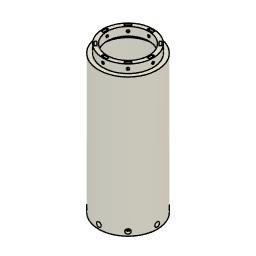
section_fuselage_basique v7 (Autodesk Fusion 360 design; units mm, degrees)
Autodesk Fusion 360 part; units mm, degrees
note: some values were not read from the file. Chosen so that the rebuilt part matches the saved one: which pieces of a blend or face edit are solid.
sketch "Esquisse1" plane through (0, 0, 0) normal (0, 1, 0) x (1, 0, 0)
  circle A0 centre (0, 0) radius 35
  circle A1 centre (0, 0) radius 30
  dimension "d1" = 70
  dimension "d2" = 60
  constraint coincident A0.centre A1.centre
  measures "d1" diameter of A0
  measures "d2" diameter of A1
extrude "Extrusion1" add sketch "Esquisse1" along normal mid plane 150 makes body 1
sketch "Esquisse1 (2)" plane through (0, 0, 0) normal (0, 1, 0) x (1, 0, 0) in component "couplage_standard_femelle v8"
  circle A0 centre (0, 0) radius 35
  circle A1 centre (0, 0) radius 30
  dimension "d1_1" = 70
  dimension "d2_1" = 60
  constraint coincident A0.centre A1.centre
  constraint concentric A0 A1
  measures "d1_1" diameter of A0
  measures "d2_1" diameter of A1
extrude "Extrusion1'" add sketch "Esquisse1 (2)" along normal mid plane 10 separate body makes body 2 in component "couplage_standard_femelle v8"
ref_plane "Plan de construction1" through (35, 0, 0) normal (1, 0, 0) x (0, 1, 0) in component "couplage_standard_femelle v8"
ref_plane "Plan de construction2" through (-35, 0, 0) normal (1, 0, 0) x (0, 1, 0) in component "couplage_standard_femelle v8"
ref_plane "Plan de construction3" through (0, 0, 35) normal (0, 0, 1) x (1, 0, 0) in component "couplage_standard_femelle v8"
ref_plane "Plan de construction4" through (0, 0, -35) normal (0, 0, 1) x (1, 0, 0) in component "couplage_standard_femelle v8"
sketch "Esquisse2" plane through (35, 0, 0) normal (1, 0, 0) x (0, 0, -1) in component "couplage_standard_femelle v8"
  circle A0 centre (0, 0) radius 1.5
  circle A1 centre (0, 0) radius 2.25
  dimension "d9" = 3
  dimension "d10" = 4.5
  constraint coincident A0.centre A1.centre
  constraint concentric A0 A1
  measures "d9" diameter of A0
  measures "d10" diameter of A1
extrude "Extrusion2" cut sketch "Esquisse2" against normal blind 70 contours A0 bodies 2 in component "couplage_standard_femelle v8"
extrude "Extrusion3" cut sketch "Esquisse2" against normal blind 3 bodies 2 in component "couplage_standard_femelle v8"
sketch "Esquisse3" plane through (-35, 0, 0) normal (1, 0, 0) x (0, 0, -1) in component "couplage_standard_femelle v8"
  circle A0 centre (0, 0) radius 2.25
  circle A1 centre (0, 0) radius 1.5
extrude "Extrusion4" cut sketch "Esquisse3" along normal blind 3 bodies 2 in component "couplage_standard_femelle v8"
sketch "Esquisse4" plane through (0, 0, 35) normal (0, 0, 1) x (1, 0, 0) in component "couplage_standard_femelle v8"
  circle A0 centre (0, 0) radius 1.5
  circle A1 centre (0, 0) radius 2.25
  dimension "d17" = 3
  dimension "d18" = 4.5
  constraint coincident A0.centre A1.centre
  measures "d17" diameter of A0
  measures "d18" diameter of A1
extrude "Extrusion5" cut sketch "Esquisse4" against normal blind 70 contours A0 bodies 2 in component "couplage_standard_femelle v8"
extrude "Extrusion6" cut sketch "Esquisse4" against normal blind 3 bodies 2 in component "couplage_standard_femelle v8"
sketch "Esquisse5" plane through (0, 0, -35) normal (0, 0, 1) x (1, 0, 0) in component "couplage_standard_femelle v8"
  circle A0 centre (0, 0) radius 1.5
  circle A1 centre (0, 0) radius 2.25
extrude "Extrusion7" cut sketch "Esquisse5" along normal blind 3 bodies 2 in component "couplage_standard_femelle v8"
move_body "Déplacer1" bodies 2 to x (0.707107, 0, 0.707107) y (0, 1, 0) z (-0.707107, 0, 0.707107) at (0, 0, 0) in component "couplage_standard_femelle v8"
ref_plane "Plan de construction5" through (35, 0, 0) normal (1, 0, 0) x (0, 1, 0) in component "couplage_standard_femelle v8"
ref_plane "Plan de construction6" through (-35, 0, 0) normal (1, 0, 0) x (0, 1, 0) in component "couplage_standard_femelle v8"
ref_plane "Plan de construction7" through (0, 0, 35) normal (0, 0, 1) x (1, 0, 0) in component "couplage_standard_femelle v8"
ref_plane "Plan de construction8" through (0, 0, -35) normal (0, 0, 1) x (1, 0, 0) in component "couplage_standard_femelle v8"
extrude "Extrusion8" cut sketch "Esquisse4" against normal blind 70 contours A0 bodies 2 in component "couplage_standard_femelle v8"
extrude "Extrusion9" cut sketch "Esquisse4" against normal blind 3 bodies 2 in component "couplage_standard_femelle v8"
sketch "Esquisse6" plane through (0, 0, -35) normal (0, 0, 1) x (1, 0, 0) in component "couplage_standard_femelle v8"
  circle A0 centre (0, 0) radius 2.25
  circle A1 centre (0, 0) radius 1.5
extrude "Extrusion10" cut sketch "Esquisse6" along normal blind 3 bodies 2 in component "couplage_standard_femelle v8"
sketch "Esquisse7" plane through (-35, 0, 0) normal (1, 0, 0) x (0, 0, -1) in component "couplage_standard_femelle v8"
  circle A0 centre (0, 0) radius 1.5
  circle A1 centre (0, 0) radius 2.25
  dimension "d35" = 3
  dimension "d36" = 4.5
  constraint coincident A0.centre A1.centre
  measures "d35" diameter of A0
  measures "d36" diameter of A1
extrude "Extrusion11" cut sketch "Esquisse7" along normal blind 70 contours A0 bodies 2 in component "couplage_standard_femelle v8"
extrude "Extrusion12" cut sketch "Esquisse7" along normal blind 3 bodies 2 in component "couplage_standard_femelle v8"
sketch "Esquisse8" plane through (35, 0, 0) normal (1, 0, 0) x (0, 0, -1) in component "couplage_standard_femelle v8"
  circle A0 centre (0, 0) radius 2.25
  circle A1 centre (0, 0) radius 1.5
extrude "Extrusion13" cut sketch "Esquisse8" against normal blind 3 bodies 2 in component "couplage_standard_femelle v8"
move_face "DécalerLesFaces1" offset -0.5 8 faces at (23.3345, 2.25, 23.3345) (33, 2.25, 0) (23.3345, 2.25, -23.3345) (0, 2.25, -33) (-23.3345, 2.25, -23.3345) (-33, 2.25, 0) (-23.3345, 2.25, 23.3345) (0, 2.25, 33) on bodies 2 in component "couplage_standard_femelle v8"
combine "Combiner1" operation add target body 1 tool bodies 2 body 2 seen with x (1, 0, 0) y (0, 1, 0) z (0, 0, 1) at (0, -80, 0)
sketch "Esquisse1 (3)" plane through (0, 0, 0) normal (0, 1, 0) x (1, 0, 0) in component "couplage_standard_male v8"
  circle A0 centre (0, 0) radius 30
  circle A1 centre (0, 0) radius 25
  dimension "d1_2" = 60
  constraint coincident A0.centre A1.centre
  constraint concentric A0 A1
  measures "d1_2" diameter of A0
extrude "Extrusion1''" add sketch "Esquisse1 (3)" along normal mid plane 10 separate body makes body 3 in component "couplage_standard_male v8"
sketch "Esquisse2 (2)" plane through (0, -5, 0) normal (0, -1, 0) x (1, 0, 0) in component "couplage_standard_male v8"
  circle A0 centre (0, 0) radius 25
  circle A1 centre (0, 0) radius 30
  circle A2 centre (0, 0) radius 35
  dimension "d4_2" = 70
  constraint coincident A0.centre A1.centre
  measures "d4_2" diameter of A2
extrude "Extrusion2'" add sketch "Esquisse2 (2)" along normal blind 5 contours A1 | A2 bodies 3 in component "couplage_standard_male v8"
ref_plane "Plan de construction1" through (30, 0, 0) normal (1, 0, 0) x (0, 1, 0) in component "couplage_standard_male v8"
ref_plane "Plan de construction2" through (-30, 0, 0) normal (1, 0, 0) x (0, 1, 0) in component "couplage_standard_male v8"
ref_plane "Plan de construction3" through (0, 0, 30) normal (0, 0, 1) x (1, 0, 0) in component "couplage_standard_male v8"
ref_plane "Plan de construction4" through (0, 0, -30) normal (0, 0, 1) x (1, 0, 0) in component "couplage_standard_male v8"
sketch "Esquisse3 (2)" plane through (30, 0, 0) normal (1, 0, 0) x (0, 0, -1) in component "couplage_standard_male v8"
  circle A0 centre (0, 0) radius 1.5
  dimension "d11_1" = 3
  constraint coincident A0.centre origin
  measures "d11_1" diameter of A0
extrude "Extrusion3'" cut sketch "Esquisse3 (2)" against normal blind 60 bodies 3 in component "couplage_standard_male v8"
sketch "Esquisse4 (2)" plane through (0, 0, -30) normal (0, 0, 1) x (1, 0, 0) in component "couplage_standard_male v8"
  circle A0 centre (0, 0) radius 1.5
  dimension "d14_1" = 3
  constraint coincident A0.centre origin
  measures "d14_1" diameter of A0
extrude "Extrusion4'" cut sketch "Esquisse4 (2)" along normal blind 60 bodies 3 in component "couplage_standard_male v8"
sketch "Esquisse5 (2)" plane through (0, 5, 0) normal (0, 1, 0) x (-1, 0, 0) in component "couplage_standard_male v8"
  circle A0 centre (0, 0) radius 25
  circle A1 centre (0, 0) radius 30
  line L0 (0, 30) -> (0, 25) construction
  line L1 (0, 27.5) -> (-5, 27.5) construction
  line L2 (0, 27.5) -> (5, 27.5) construction
  line L3 (0, 27.5) -> (0, 26.25)
  line L4 (0, 27.5) -> (0, 28.75)
  line L5 (0, 26.25) -> (3.25, 26.25)
  line L6 (0, 28.75) -> (3.25, 28.75)
  line L7 (3.25, 28.75) -> (3.25, 26.25)
  line L8 (0, 26.25) -> (-3.25, 26.25)
  line L9 (0, 28.75) -> (-3.25, 28.75)
  line L10 (-3.25, 28.75) -> (-3.25, 26.25)
  line L11 (-18.5616, 18.5616) -> (-16.2635, 20.8597)
  line L12 (-19.4454, 19.4454) -> (-18.5616, 18.5616)
  line L13 (-19.4454, 19.4454) -> (-20.3293, 20.3293)
  line L14 (-20.3293, 20.3293) -> (-18.0312, 22.6274)
  line L15 (-18.0312, 22.6274) -> (-16.2635, 20.8597)
  line L16 (-18.5616, 18.5616) -> (-20.8597, 16.2635)
  line L17 (-22.6274, 18.0312) -> (-20.8597, 16.2635)
  line L18 (-20.3293, 20.3293) -> (-22.6274, 18.0312)
  line L19 (-19.4454, 19.4454) -> (-22.981, 15.9099) construction
  line L20 (-19.4454, 19.4454) -> (-15.9099, 22.981) construction
  line L21 (-21.2132, 21.2132) -> (-17.6777, 17.6777) construction
  line L22 (-26.25, 0) -> (-26.25, 3.25)
  line L23 (-27.5, 0) -> (-26.25, 0)
  line L24 (-27.5, 0) -> (-28.75, 0)
  line L25 (-28.75, 0) -> (-28.75, 3.25)
  line L26 (-28.75, 3.25) -> (-26.25, 3.25)
  line L27 (-26.25, 0) -> (-26.25, -3.25)
  line L28 (-28.75, -3.25) -> (-26.25, -3.25)
  line L29 (-28.75, 0) -> (-28.75, -3.25)
  line L30 (-27.5, 0) -> (-27.5, -5) construction
  line L31 (-27.5, 0) -> (-27.5, 5) construction
  line L32 (-30, 0) -> (-25, 0) construction
  line L33 (-18.5616, -18.5616) -> (-20.8597, -16.2635)
  line L34 (-19.4454, -19.4454) -> (-18.5616, -18.5616)
  line L35 (-19.4454, -19.4454) -> (-20.3293, -20.3293)
  line L36 (-20.3293, -20.3293) -> (-22.6274, -18.0312)
  line L37 (-22.6274, -18.0312) -> (-20.8597, -16.2635)
  line L38 (-18.5616, -18.5616) -> (-16.2635, -20.8597)
  line L39 (-18.0312, -22.6274) -> (-16.2635, -20.8597)
  line L40 (-20.3293, -20.3293) -> (-18.0312, -22.6274)
  line L41 (-19.4454, -19.4454) -> (-15.9099, -22.981) construction
  line L42 (-19.4454, -19.4454) -> (-22.981, -15.9099) construction
  line L43 (-21.2132, -21.2132) -> (-17.6777, -17.6777) construction
  line L44 (0, -26.25) -> (-3.25, -26.25)
  line L45 (0, -27.5) -> (0, -26.25)
  line L46 (0, -27.5) -> (0, -28.75)
  line L47 (0, -28.75) -> (-3.25, -28.75)
  line L48 (-3.25, -28.75) -> (-3.25, -26.25)
  line L49 (0, -26.25) -> (3.25, -26.25)
  line L50 (3.25, -28.75) -> (3.25, -26.25)
  line L51 (0, -28.75) -> (3.25, -28.75)
  line L52 (0, -27.5) -> (5, -27.5) construction
  line L53 (0, -27.5) -> (-5, -27.5) construction
  line L54 (0, -30) -> (0, -25) construction
  line L55 (18.5616, -18.5616) -> (16.2635, -20.8597)
  line L56 (19.4454, -19.4454) -> (18.5616, -18.5616)
  line L57 (19.4454, -19.4454) -> (20.3293, -20.3293)
  line L58 (20.3293, -20.3293) -> (18.0312, -22.6274)
  line L59 (18.0312, -22.6274) -> (16.2635, -20.8597)
  line L60 (18.5616, -18.5616) -> (20.8597, -16.2635)
  line L61 (22.6274, -18.0312) -> (20.8597, -16.2635)
  line L62 (20.3293, -20.3293) -> (22.6274, -18.0312)
  line L63 (19.4454, -19.4454) -> (22.981, -15.9099) construction
  line L64 (19.4454, -19.4454) -> (15.9099, -22.981) construction
  line L65 (21.2132, -21.2132) -> (17.6777, -17.6777) construction
  line L66 (26.25, 0) -> (26.25, -3.25)
  line L67 (27.5, 0) -> (26.25, 0)
  line L68 (27.5, 0) -> (28.75, 0)
  line L69 (28.75, 0) -> (28.75, -3.25)
  line L70 (28.75, -3.25) -> (26.25, -3.25)
  line L71 (26.25, 0) -> (26.25, 3.25)
  line L72 (28.75, 3.25) -> (26.25, 3.25)
  line L73 (28.75, 0) -> (28.75, 3.25)
  line L74 (27.5, 0) -> (27.5, 5) construction
  line L75 (27.5, 0) -> (27.5, -5) construction
  line L76 (30, 0) -> (25, 0) construction
  line L77 (18.5616, 18.5616) -> (20.8597, 16.2635)
  line L78 (19.4454, 19.4454) -> (18.5616, 18.5616)
  line L79 (19.4454, 19.4454) -> (20.3293, 20.3293)
  line L80 (20.3293, 20.3293) -> (22.6274, 18.0312)
  line L81 (22.6274, 18.0312) -> (20.8597, 16.2635)
  line L82 (18.5616, 18.5616) -> (16.2635, 20.8597)
  line L83 (18.0312, 22.6274) -> (16.2635, 20.8597)
  line L84 (20.3293, 20.3293) -> (18.0312, 22.6274)
  line L85 (19.4454, 19.4454) -> (15.9099, 22.981) construction
  line L86 (19.4454, 19.4454) -> (22.981, 15.9099) construction
  line L87 (21.2132, 21.2132) -> (17.6777, 17.6777) construction
  dimension "d17_1" = 1.25
  dimension "d18_1" = 1.25
  dimension "d19_1" = 3.25
  dimension "d20_1" = 3.25
  dimension "d21_1" = 3.25
  dimension "d25_1" = 360
  constraint coincident A1 L0.start
  constraint coincident A0 L0.end
  constraint vertical L0
  constraint midpoint L0 L1.start
  constraint perpendicular L0 L1
  constraint perpendicular L0 L2
  constraint coincident L0 L3.end
  constraint perpendicular L1 L4
  constraint perpendicular L3 L5
  constraint perpendicular L4 L6
  constraint perpendicular L3 L8
  constraint perpendicular L0 L9
  constraint perpendicular L8 L10
  measures "d17_1" distance of L1.start L3.end
  measures "d18_1" distance of L1.start L4.end
  measures "d19_1" distance of L3.end L5.end
  measures "d20_1" distance of L4.end L6.end
  measures "d21_1" distance of L3.end L8.end
extrude "Extrusion6'" cut sketch "Esquisse5 (2)" against normal blind 8 contours L3 L4 L5 L6 L7 | L3 L4 L8 L9 L10 | L11 L12 L13 L14 L15 | L12 L13 L16 L17 L18 | L22 L23 L24 L25 L26 | L23 L24 L27 L28 L29 | L33 L34 L35 L36 L37 | L34 L35 L38 L39 L40 | L44 L45 L46 L47 L48 | L45 L46 L49 L50 L51 | L55 L56 L57 L58 L59 | L56 L57 L60 L61 L62 | L66 L67 L68 L69 L70 | L67 L68 L71 L72 L73 | L77 L78 L79 L80 L81 | L78 L79 L82 L83 L84 bodies 3 in component "couplage_standard_male v8"
move_body "Déplacer1'" bodies 3 to x (0.707107, 0, 0.707107) y (0, 1, 0) z (-0.707107, 0, 0.707107) at (0, 0, 0) in component "couplage_standard_male v8"
ref_plane "Plan de construction5" through (0, 0, -30) normal (0, 0, 1) x (1, 0, 0) in component "couplage_standard_male v8"
ref_plane "Plan de construction6" through (30, 0, 0) normal (1, 0, 0) x (0, 1, 0) in component "couplage_standard_male v8"
sketch "Esquisse6 (2)" plane through (30, 0, 0) normal (1, 0, 0) x (0, 0, -1) in component "couplage_standard_male v8"
  circle A0 centre (0, 0) radius 1.5
  dimension "d30_1" = 3
  constraint coincident A0.centre origin
  measures "d30_1" diameter of A0
sketch "Esquisse7 (2)" plane through (0, 0, -30) normal (0, 0, 1) x (1, 0, 0) in component "couplage_standard_male v8"
  circle A0 centre (0, 0) radius 1.5
  dimension "d31_1" = 3
  constraint coincident A0.centre origin
  measures "d31_1" diameter of A0
extrude "Extrusion7'" cut sketch "Esquisse6 (2)" against normal blind 60 bodies 3 in component "couplage_standard_male v8"
extrude "Extrusion8'" cut sketch "Esquisse7 (2)" along normal blind 60 bodies 3 in component "couplage_standard_male v8"
chamfer "Chanfrein1" distance 5 angle 45 1 edges at (-22.8739, -10, -10.0889) on bodies 3 in component "couplage_standard_male v8"
combine "Combiner2" operation add target body 1 tool bodies 3 body 3 seen with x (1, 0, 0) y (0, 1, 0) z (0, 0, 1) at (0, 85, 0)
extrude "Extrusion2''" cut 1 faces at (24.1493, -80.8849, 21.1055) along direction (-0.707107, 0, -0.707107) blind 1 on bodies 1 bodies 1
extrude "Extrusion3''" cut 1 faces at (32, -80.8849, -2.1523) along direction (-1, 0, 0) blind 1 on bodies 1 bodies 1
extrude "Extrusion4''" cut 1 faces at (24.1493, -80.8849, -21.1055) along direction (-0.707107, 0, 0.707107) blind 1 on bodies 1 bodies 1
extrude "Extrusion5'" cut 1 faces at (-2.1796, -80.8153, -32) along direction (0, 0, 1) blind 1 on bodies 1 bodies 1
extrude "Extrusion6''" cut 1 faces at (-21.1055, -80.8849, -24.1493) along direction (0.707107, 0, 0.707107) blind 1 on bodies 1 bodies 1
extrude "Extrusion7''" cut 1 faces at (-32, -80.8849, -2.1523) along direction (1, 0, 0) blind 1 on bodies 1 bodies 1
extrude "Extrusion8''" cut 1 faces at (-21.1055, -80.8849, 24.1493) along direction (0.707107, 0, -0.707107) blind 1 on bodies 1 bodies 1
extrude "Extrusion9'" cut 1 faces at (-2.1796, -80.8153, 32) along direction (0, 0, -1) blind 1 on bodies 1 bodies 1
ref_plane "Plan de construction1" through (0, -75, 0) normal (0, 1, 0) x (0, 0, 1)
split "Scinder1" by plane through (0, -75, 0) normal (0, 1, 0) bodies 1 makes body 4 at (31.9027, 28.3333, 14.395)
move_face "DécalerLesFaces1'" offset -0.5 1 faces at (-29.4263, -80.0323, 5.8392) on bodies 1
combine "Combiner3" operation add target body 4 tool bodies 1
component "couplage_standard_femelle v8" placed x (1, 0, 0) y (0, 1, 0) z (0, 0, 1) at (0, -80, 0)
component "couplage_standard_male v8" placed x (1, 0, 0) y (0, 1, 0) z (0, 0, 1) at (0, 85, 0)
equation "d17_1 = ( 2.5 / 2 ) * 1 mm"
equation "d18_1 = ( 2.5 / 2 ) * 1 mm"
equation "d19_1 = ( 6.5 / 2 ) * 1 mm"
equation "d20_1 = ( 6.5 / 2 ) * 1 mm"
equation "d21_1 = ( 6.5 / 2 ) * 1 mm"
named bodies: "section_fuselage", "section_fuselage (1)"
